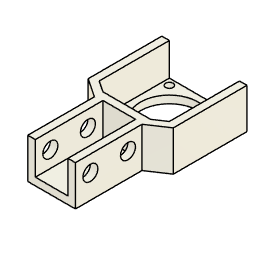
LinkExtender (Autodesk Fusion 360 design; units mm, degrees)
Autodesk Fusion 360 part; units mm, degrees
sketch "Sketch1" plane through (0, 0, 0) normal (1, 0, 0) x (0, 1, 0)
  line L0 (0, 0) -> (27, 0)
  line L1 (27, 0) -> (27, 16)
  line L2 (27, 16) -> (0, 16)
  line L3 (0, 16) -> (0, 0)
  line L4 (0, 9.5) -> (6, 9.5) construction
  line L5 (6, 9.5) -> (6, 16) construction
  circle A0 centre (6, 9.5) radius 3
  line L6 (6, 9.5) -> (21, 9.5)
  circle A1 centre (21, 9.5) radius 3
  dimension "d1_4" = 16
  dimension "d2_4" = 27
  dimension "d3_4" = 6
  dimension "d4_4" = 6.5
  dimension "d5_2" = 6
  dimension "d6_1" = 15
  dimension "d7_2" = 6
  constraint horizontal L0
  constraint vertical L1
  constraint horizontal L2
  constraint vertical L3
  constraint coincident L0.start L3.end
  constraint perpendicular L3 L4
  constraint coincident L2 L5.end
  constraint perpendicular L2 L5
  constraint coincident L3 L4.start
  constraint coincident L4.end L5.start
  constraint perpendicular L5 L6
  constraint coincident L6.end A1.centre
  measures "d1_4" distance of L0.start L2.end
  measures "d2_4" distance of L1.end L2.end
  measures "d3_4" distance of L4.start L4.end
  measures "d4_4" distance of L4.end L5.end
  measures "d5_2" diameter of A0
  measures "d6_1" distance of L4.end L6.end
  measures "d7_2" diameter of A1
extrude "Extrude1" add sketch "Sketch1" along normal blind 3 makes body 1
sketch "Sketch2" plane through (0, 0, 0) normal (-1, 0, 0) x (0, -1, 0)
  circle A0 centre (-21, 9.5) radius 3
  circle A1 centre (-6, 9.5) radius 3
  line L0 (0, 0) -> (0, 16)
  line L1 (0, 16) -> (-27, 16)
  line L2 (-27, 16) -> (-27, 0)
  line L3 (-27, 0) -> (0, 0)
  line L4 (0, 0) -> (-27, 0)
  line L5 (-27, 0) -> (-27, 3)
  line L6 (-27, 3) -> (0, 3)
  line L7 (0, 3) -> (0, 0)
  dimension "d10_1" = 3
  constraint horizontal L4
  constraint vertical L5
  constraint horizontal L6
  constraint vertical L7
  constraint coincident L2 L5.end
  constraint coincident L0.start L3.end
  measures "d10_1" distance of L0.start L6.end
extrude "Extrude2" add sketch "Sketch2" along normal blind 13 contours L0 L2 L3 L4 L5 L6 L7 bodies 1
ref_plane "WorkPlane1" through (-6.5, 13.5, 1.5) normal (-1, 0, 0) x (0, 0, 1)
mirror "Mirror1" about plane through (-6.5, 13.5, 1.5) normal (-1, 0, 0) of "Extrude1" makes body 2
combine "Combine1" operation add target body 1 tool bodies 2
sketch "Sketch3" plane through (0, 27, 0) normal (0, 1, 0) x (-1, 0, 0)
  line L0 (0, 3) -> (0, 16)
  line L1 (0, 16) -> (-3, 16)
  line L2 (-3, 16) -> (-3, 0)
  line L3 (-3, 0) -> (16, 0)
  line L4 (16, 0) -> (16, 16)
  line L5 (16, 16) -> (13, 16)
  line L6 (13, 16) -> (13, 3)
  line L7 (13, 3) -> (0, 3)
  line L8 (-3, 16) -> (16, 16)
  line L9 (16, 16) -> (16, 0)
  line L10 (16, 0) -> (-3, 0)
  line L11 (-3, 0) -> (-3, 16)
  constraint horizontal L8
  constraint vertical L9
  constraint horizontal L10
  constraint vertical L11
  constraint coincident L3.end L4.start
  constraint coincident L1.end L2.start
extrude "Extrude3" add sketch "Sketch3" along normal blind 3 bodies 1
sketch "Sketch4" plane through (0, 0, 0) normal (0, 0, -1) x (1, 0, 0)
  line L0 (3, -30) -> (3, 0)
  line L1 (3, 0) -> (-16, 0)
  line L2 (-16, 0) -> (-16, -30)
  line L3 (-16, -30) -> (3, -30)
  line L4 (-6.5, -30) -> (-6.5, -33) construction
  line L5 (7.5, -33) -> (-20.5, -33) construction
  line L6 (-20.5, -33) -> (-20.5, -61)
  line L7 (-20.5, -61) -> (7.5, -61)
  line L8 (7.5, -61) -> (7.5, -33)
  line L9 (-16, -30) -> (-20.5, -33)
  line L10 (3, -30) -> (7.5, -33)
  circle A0 centre (-6.5, -47) radius 11.5
  line L11 (7.5, -33) -> (-20.5, -61) construction
  line L12 (7.5, -61) -> (-20.5, -33) construction
  dimension "d23" = 28
  dimension "d24" = 28
  dimension "d25" = 3
  dimension "d28" = 23
  constraint midpoint L3 L4.start
  constraint perpendicular L3 L4
  constraint horizontal L5
  constraint vertical L6
  constraint horizontal L7
  constraint vertical L8
  constraint coincident L4.end L5
  constraint midpoint L4.end L5
  constraint coincident L2.end L3.start
  constraint coincident L0.start L3.end
  constraint midpoint A0.centre L11
  measures "d23" distance of L5.start L5.end
  measures "d24" distance of L5.start L7.end
  measures "d25" distance of L4.start L4.end
  measures "d28" diameter of A0
extrude "Extrude4" add sketch "Sketch4" against normal blind 3 contours L3 L6 L7 L8 L9 L10 bodies 1
sketch "Sketch5" plane through (0, 0, 0) normal (0, 0, -1) x (1, 0, 0)
  circle A0 centre (-6.5, -47) radius 11.5
  line L0 (3, -30) -> (3, 0)
  line L1 (3, 0) -> (-16, 0)
  line L2 (-16, 0) -> (-16, -30)
  line L3 (-16, -30) -> (-20.5, -33)
  line L4 (-20.5, -33) -> (-20.5, -61)
  line L5 (-20.5, -61) -> (7.5, -61)
  line L6 (7.5, -61) -> (7.5, -33)
  line L7 (7.5, -33) -> (3, -30)
  line L8 (7.5, -61) -> (-20.5, -61)
  line L9 (-20.5, -61) -> (-20.5, -33)
  line L10 (-20.5, -33) -> (7.5, -33)
  line L11 (7.5, -33) -> (7.5, -61)
  line L12 (5, -58.5) -> (-18, -58.5) construction
  line L13 (-18, -58.5) -> (-18, -35.5) construction
  line L14 (-18, -35.5) -> (5, -35.5) construction
  line L15 (5, -35.5) -> (5, -58.5) construction
  circle A1 centre (5, -58.5) radius 1.5
  circle A2 centre (-18, -58.5) radius 1.5
  circle A3 centre (5, -35.5) radius 1.5
  circle A4 centre (-18, -35.5) radius 1.5
  dimension "d29" = 23
  dimension "d30" = 23
  dimension "d31" = 2.5
  dimension "d32" = 2.5
  dimension "d33" = 2.5
  dimension "d34" = 2.5
  dimension "d35" = 3
  dimension "d36" = 3
  dimension "d37" = 3
  dimension "d38" = 3
  constraint horizontal L8
  constraint vertical L9
  constraint horizontal L10
  constraint vertical L11
  constraint coincident L3.end L4.start
  constraint coincident L5.end L6.start
  constraint horizontal L12
  constraint vertical L13
  constraint horizontal L14
  constraint vertical L15
  constraint coincident L12.start L15.end
  constraint coincident L12.end L13.start
  constraint coincident L14.end L15.start
  constraint coincident L13.end L14.start
  measures "d29" distance of L12.start L12.end
  measures "d30" distance of L12.start L14.end
  measures "d31" distance of L11 L15
  measures "d32" distance of L9 L13
  measures "d33" distance of L8 L12
  measures "d34" distance of L10 L14
  measures "d35" diameter of A1
  measures "d36" diameter of A2
  measures "d37" diameter of A3
  measures "d38" diameter of A4
extrude "Extrude5" cut sketch "Sketch5" against normal up to surface (3 mm away) contours A1 | A2 | A3 | A4 bodies 1
sketch "Sketch10" plane through (0, 0, 3) normal (0, 0, 1) x (-1, 0, 0)
  circle A0 centre (-5, -35.5) radius 1.5
  circle A1 centre (18, -35.5) radius 1.5
  circle A2 centre (-5, -58.5) radius 1.5
  circle A3 centre (18, -58.5) radius 1.5
  circle A4 centre (6.5, -47) radius 11.5
  line L0 (20.5, -33) -> (16, -30)
  line L1 (16, -30) -> (-3, -30)
  line L2 (-3, -30) -> (-7.5, -33)
  line L3 (-7.5, -33) -> (-7.5, -61)
  line L4 (-7.5, -61) -> (20.5, -61)
  line L5 (20.5, -61) -> (20.5, -33)
  line L6 (-7.5, -61) -> (-10.5, -61)
  line L7 (-10.5, -61) -> (-10.5, -33)
  line L8 (-3, -26.5806) -> (-10.5, -31.5806)
  line L9 (-10.5, -31.5806) -> (-10.5, -61)
  line L10 (-3, 0) -> (-3, -30)
  line L11 (-7.5, -61) -> (-7.5, -61)
  dimension "d91" = 3
  constraint coincident L3.end L4.start
  constraint perpendicular L3 L6
  constraint perpendicular L6 L7
  constraint coincident L8.start L10
  constraint equal L3 L7
  measures "d91" distance of L3.end L6.end
extrude "Extrude8" add sketch "Sketch10" along normal up to surface (13 mm away) and the other way up to surface (3 mm away) contours L2 L3 L6 L7 L8 L9 L10 bodies 1
mirror "Mirror3" about plane through (-6.5, 13.5, 1.5) normal (-1, 0, 0) of "Extrude8"
